Autodesk Inventor part; units mm, degrees
(part 2 of 2)
  measures "d98" distance between parallel lines of L25 L67
  measures "d99" distance between parallel lines of L23 L68
  measures "d100" distance edge to line of A24 L66
  measures "d101" radius of A116
extrude "押し出し11" cut sketch "肉抜き" against normal blind 2.5 contours A83 A92 A85 A96 L51 A97 A86 A95 A88 L53 A94 L52 A93 L50 A90 L49 A91 L48 | A98 L55 A103 L56 A102 L57 A105 L59 A106 L60 A101 A107 A100 A109 L58 A108 A99 A104 | A114 A121 A115 A120 L66 A119 L67 A118 L68 A116 L65 A117 | A126 A129 L75 A128 L78 A130 L77 A131 L76 A132 A127 A133 | A138 A141 L81 A140 L84 A142 L83 A143 L82 A144 A139 A145 | L90 A157 A156 A154 A155 A153 L89 A152 L88 A151 L87 A150 | A158 L91 A163 L92 A162 L93 A165 L95 A166 L96 A161 A167 A160 A169 L94 A168 A159 A164 | A171 L98 A172 A181 A180 A179 L102 A178 A177 A176 A175 L101 A174 L100 A173 L99 A170 L97
